Autodesk Inventor part; units mm, degrees
(part 6 of 16)
  spline S32 degree 3 poles (-26.5584, 48.5928) (-26.5078, 48.7178) (-26.4553, 48.842) (-26.4009, 48.9654) (-26.3715, 49.0321) (-26.3415, 49.0986) (-26.3109, 49.1648) (-26.2819, 49.2274) (-26.2524, 49.2898) (-26.2223, 49.3519) (-26.1939, 49.4105) (-26.165, 49.4689) (-26.1356, 49.527) (-26.1079, 49.5817) (-26.0798, 49.6361) (-26.0511, 49.6902) (-26.0243, 49.7409) (-25.997, 49.7914) (-25.9693, 49.8416) (-25.9435, 49.8884) (-25.9172, 49.935) (-25.8905, 49.9814) (-25.8658, 50.0244) (-25.8407, 50.0671) (-25.8152, 50.1097) (-25.7917, 50.1489) (-25.7679, 50.1879) (-25.7437, 50.2267) (-25.7216, 50.2622) (-25.6991, 50.2974) (-25.6764, 50.3325) (-25.6557, 50.3644) (-25.6348, 50.396) (-25.6136, 50.4275) (-25.5946, 50.4557) (-25.5753, 50.4838) (-25.5558, 50.5116) (-25.5299, 50.5485) (-25.5036, 50.5849) (-25.4769, 50.6212) (-25.4709, 50.6293) (-25.465, 50.6374) (-25.4591, 50.6456) (-25.4533, 50.6535) (-25.4476, 50.6616) (-25.442, 50.6697) (-25.4366, 50.6776) (-25.4311, 50.6855) (-25.4258, 50.6935) (-25.4205, 50.7014) (-25.4154, 50.7093) (-25.4103, 50.7172) (-25.4053, 50.725) (-25.4003, 50.7329) (-25.3955, 50.7408) (-25.3907, 50.7485) (-25.386, 50.7564) (-25.3815, 50.7642) (-25.3769, 50.772) (-25.3725, 50.7798) (-25.3681, 50.7877) (-25.3638, 50.7955) (-25.3596, 50.8034) (-25.3555, 50.8113) (-25.3514, 50.8192) (-25.3474, 50.8271) (-25.3435, 50.8351) (-25.3396, 50.8431) (-25.3358, 50.8512) (-25.3322, 50.8593) (-25.3285, 50.8675) (-25.3249, 50.8758) (-25.3215, 50.8841) (-25.3181, 50.8926) (-25.3148, 50.9011) (-25.3116, 50.9097) (-25.3084, 50.9185) (-25.3053, 50.9274) (-25.3024, 50.9364) (-25.2994, 50.9457) (-25.2967, 50.9551) (-25.2941, 50.9646) (-25.2914, 50.9746) (-25.289, 50.9846) (-25.2868, 50.9947) (-25.2845, 51.0055) (-25.2825, 51.0164) (-25.2808, 51.0274) (-25.279, 51.0393) (-25.2776, 51.0512) (-25.2767, 51.0632) (-25.2756, 51.0765) (-25.2751, 51.0897) (-25.2751, 51.103) (-25.2751, 51.1178) (-25.2759, 51.1326) (-25.2773, 51.1474) (-25.2789, 51.164) (-25.2815, 51.1804) (-25.2849, 51.1967) (-25.2888, 51.2151) (-25.2938, 51.2331) (-25.3, 51.2508) (-25.3069, 51.2704) (-25.3153, 51.2895) (-25.3249, 51.308) (-25.3354, 51.328) (-25.3475, 51.3472) (-25.3611, 51.3651) (-25.3742, 51.3822) (-25.3887, 51.3982) (-25.4035, 51.4138) (-25.4766, 51.4915) (-25.556, 51.5626) (-25.6317, 51.6374) (-25.7075, 51.7123) (-25.7795, 51.7908) (-25.858, 51.863) (-25.8739, 51.8776) (-25.89, 51.892) (-25.9072, 51.9048) (-25.9253, 51.9183) (-25.9447, 51.9301) (-25.9648, 51.9403) (-25.9833, 51.9498) (-26.0026, 51.9579) (-26.0223, 51.9646) (-26.04, 51.9706) (-26.0581, 51.9754) (-26.0765, 51.9791) (-26.0928, 51.9823) (-26.1093, 51.9847) (-26.1259, 51.9861) (-26.1407, 51.9874) (-26.1555, 51.9879) (-26.1703, 51.9878) (-26.1836, 51.9876) (-26.1969, 51.9869) (-26.2101, 51.9857) (-26.2221, 51.9846) (-26.234, 51.9831) (-26.2459, 51.9812) (-26.2568, 51.9794) (-26.2677, 51.9772) (-26.2785, 51.9748) (-26.2885, 51.9725) (-26.2986, 51.97) (-26.3085, 51.9672) (-26.318, 51.9645) (-26.3273, 51.9616) (-26.3366, 51.9585) (-26.3455, 51.9555) (-26.3544, 51.9524) (-26.3632, 51.949) (-26.3718, 51.9458) (-26.3802, 51.9423) (-26.3887, 51.9388) (-26.3969, 51.9353) (-26.4052, 51.9316) (-26.4133, 51.9279) (-26.4214, 51.9241) (-26.4294, 51.9202) (-26.4374, 51.9163) (-26.4453, 51.9123) (-26.4532, 51.9082) (-26.4611, 51.904) (-26.4689, 51.8998) (-26.4767, 51.8955) (-26.4845, 51.8911) (-26.4923, 51.8866) (-26.5001, 51.8821) (-26.5078, 51.8775) (-26.5156, 51.8728) (-26.5234, 51.868) (-26.5311, 51.8631) (-26.539, 51.8582) (-26.5468, 51.8532) (-26.5545, 51.8481) (-26.5624, 51.8429) (-26.5702, 51.8376) (-26.578, 51.8323) (-26.5859, 51.8269) (-26.5938, 51.8213) (-26.6017, 51.8158) (-26.6097, 51.8101) (-26.6177, 51.8043) (-26.6256, 51.7984) (-26.6337, 51.7925) (-26.6417, 51.7864) (-26.6497, 51.7803) (-26.6857, 51.7532) (-26.7218, 51.7265) (-26.7583, 51.7002) (-26.786, 51.6803) (-26.8138, 51.6607) (-26.8418, 51.6414) (-26.8731, 51.6198) (-26.9045, 51.5985) (-26.936, 51.5775) (-26.9708, 51.5543) (-27.0059, 51.5315) (-27.0411, 51.5089) (-27.0796, 51.4843) (-27.1183, 51.46) (-27.1572, 51.436) (-27.1995, 51.41) (-27.2419, 51.3844) (-27.2846, 51.3592) (-27.3307, 51.332) (-27.377, 51.3052) (-27.4235, 51.2788) (-27.4734, 51.2505) (-27.5235, 51.2227) (-27.5739, 51.1952) (-27.6277, 51.166) (-27.6818, 51.1372) (-27.7361, 51.1089) (-27.7938, 51.0788) (-27.8519, 51.0492) (-27.9102, 51.0201) (-27.9719, 50.9893) (-28.034, 50.959) (-28.0963, 50.9293) (-28.1621, 50.898) (-28.2282, 50.8672) (-28.2945, 50.837) (-28.4173, 50.7811) (-28.5409, 50.7272) (-28.6653, 50.6751) knots 0 0 0 0 0.057795 0.057795 0.057795 0.089038 0.089038 0.089038 0.118617 0.118617 0.118617 0.14653 0.14653 0.14653 0.172778 0.172778 0.172778 0.19736 0.19736 0.19736 0.220277 0.220277 0.220277 0.241529 0.241529 0.241529 0.261115 0.261115 0.261115 0.279036 0.279036 0.279036 0.295292 0.295292 0.295292 0.309882 0.309882 0.309882 0.329164 0.329164 0.329164 0.333477 0.333477 0.333477 0.337694 0.337694 0.337694 0.34182 0.34182 0.34182 0.345864 0.345864 0.345864 0.349834 0.349834 0.349834 0.353742 0.353742 0.353742 0.3576 0.3576 0.3576 0.361424 0.361424 0.361424 0.365232 0.365232 0.365232 0.369048 0.369048 0.369048 0.372899 0.372899 0.372899 0.376819 0.376819 0.376819 0.380853 0.380853 0.380853 0.385052 0.385052 0.385052 0.389482 0.389482 0.389482 0.394225 0.394225 0.394225 0.399381 0.399381 0.399381 0.405067 0.405067 0.405067 0.411413 0.411413 0.411413 0.418548 0.418548 0.418548 0.426565 0.426565 0.426565 0.435472 0.435472 0.435472 0.445133 0.445133 0.445133 0.45436 0.45436 0.45436 0.5 0.5 0.5 0.54564 0.54564 0.54564 0.554867 0.554867 0.554867 0.564528 0.564528 0.564528 0.573435 0.573435 0.573435 0.581452 0.581452 0.581452 0.588587 0.588587 0.588587 0.594933 0.594933 0.594933 0.600619 0.600619 0.600619 0.605775 0.605775 0.605775 0.610518 0.610518 0.610518 0.614948 0.614948 0.614948 0.619147 0.619147 0.619147 0.623181 0.623181 0.623181 0.627101 0.627101 0.627101 0.630952 0.630952 0.630952 0.634768 0.634768 0.634768 0.638576 0.638576 0.638576 0.6424 0.6424 0.6424 0.646258 0.646258 0.646258 0.650166 0.650166 0.650166 0.654136 0.654136 0.654136 0.65818 0.65818 0.65818 0.662306 0.662306 0.662306 0.666523 0.666523 0.666523 0.670836 0.670836 0.670836 0.690118 0.690118 0.690118 0.704708 0.704708 0.704708 0.720964 0.720964 0.720964 0.738885 0.738885 0.738885 0.758471 0.758471 0.758471 0.779723 0.779723 0.779723 0.80264 0.80264 0.80264 0.827222 0.827222 0.827222 0.85347 0.85347 0.85347 0.881383 0.881383 0.881383 0.910962 0.910962 0.910962 0.942205 0.942205 0.942205 1 1 1 1
  arc A234 (-26.5584, 48.5928) -> (-25.692, 47.8218) centre (0.0435, 77.6158) ccw
  spline S33 degree 3 poles (-23.379, 45.9711) (-23.3417, 46.1007) (-23.3025, 46.2298) (-23.2613, 46.3582) (-23.239, 46.4276) (-23.2161, 46.4968) (-23.1926, 46.5658) (-23.1703, 46.6312) (-23.1475, 46.6963) (-23.124, 46.7612) (-23.1019, 46.8225) (-23.0793, 46.8836) (-23.0561, 46.9444) (-23.0343, 47.0017) (-23.012, 47.0587) (-22.9891, 47.1156) (-22.9678, 47.1688) (-22.9459, 47.2218) (-22.9236, 47.2747) (-22.9028, 47.324) (-22.8816, 47.373) (-22.8599, 47.4219) (-22.8398, 47.4673) (-22.8193, 47.5124) (-22.7984, 47.5574) (-22.7791, 47.5988) (-22.7595, 47.6401) (-22.7395, 47.6812) (-22.7212, 47.7188) (-22.7026, 47.7563) (-22.6836, 47.7935) (-22.6664, 47.8273) (-22.6489, 47.861) (-22.6311, 47.8945) (-22.6151, 47.9246) (-22.5989, 47.9545) (-22.5824, 47.9843) (-22.5605, 48.0236) (-22.5381, 48.0626) (-22.5154, 48.1015) (-22.5103, 48.1101) (-22.5052, 48.1188) (-22.5002, 48.1276) (-22.4953, 48.1361) (-22.4905, 48.1447) (-22.4858, 48.1533) (-22.4812, 48.1617) (-22.4766, 48.1702) (-22.4721, 48.1787) (-22.4677, 48.1871) (-22.4634, 48.1955) (-22.4592, 48.2039) (-22.455, 48.2122) (-22.4509, 48.2205) (-22.4469, 48.2289) (-22.443, 48.2371) (-22.4392, 48.2454) (-22.4354, 48.2537) (-22.4317, 48.2619) (-22.4281, 48.2701) (-22.4246, 48.2784) (-22.4211, 48.2867) (-22.4178, 48.2949) (-22.4145, 48.3032) (-22.4112, 48.3115) (-22.4081, 48.3198) (-22.4051, 48.3282) (-22.402, 48.3365) (-22.3991, 48.345) (-22.3963, 48.3534) (-22.3935, 48.362) (-22.3909, 48.3705) (-22.3884, 48.3792) (-22.3858, 48.3879) (-22.3834, 48.3968) (-22.3812, 48.4056) (-22.3789, 48.4148) (-22.3767, 48.4239) (-22.3748, 48.4332) (-22.3728, 48.4428) (-22.371, 48.4524) (-22.3695, 48.4621) (-22.3679, 48.4723) (-22.3665, 48.4825) (-22.3654, 48.4928) (-22.3642, 48.5038) (-22.3634, 48.5149) (-22.3629, 48.5259) (-22.3623, 48.5379) (-22.3622, 48.55) (-22.3625, 48.562) (-22.3628, 48.5753) (-22.3637, 48.5885) (-22.3651, 48.6017) (-22.3667, 48.6165) (-22.3689, 48.6311) (-22.3719, 48.6456) (-22.3752, 48.6619) (-22.3795, 48.6781) (-22.3846, 48.6939) (-22.3904, 48.7117) (-22.3973, 48.7292) (-22.4053, 48.7461) (-22.4142, 48.7649) (-22.4245, 48.783) (-22.4361, 48.8003) (-22.4486, 48.8191) (-22.4626, 48.837) (-22.478, 48.8534) (-22.4928, 48.869) (-22.5089, 48.8834) (-22.5253, 48.8975) (-22.6061, 48.967) (-22.6925, 49.0295) (-22.7756, 49.096) (-22.8587, 49.1625) (-22.9386, 49.2331) (-23.0242, 49.2967) (-23.0415, 49.3095) (-23.059, 49.3221) (-23.0776, 49.3331) (-23.097, 49.3446) (-23.1174, 49.3543) (-23.1385, 49.3624) (-23.1579, 49.3698) (-23.1779, 49.3759) (-23.1982, 49.3805) (-23.2164, 49.3846) (-23.235, 49.3875) (-23.2536, 49.3892) (-23.2702, 49.3908) (-23.2869, 49.3914) (-23.3035, 49.391) (-23.3183, 49.3908) (-23.3331, 49.3898) (-23.3479, 49.3881) (-23.361, 49.3865) (-23.3742, 49.3845) (-23.3872, 49.3819) (-23.399, 49.3795) (-23.4107, 49.3768) (-23.4223, 49.3736) (-23.433, 49.3707) (-23.4436, 49.3674) (-23.4541, 49.3639) (-23.4639, 49.3606) (-23.4735, 49.357) (-23.4832, 49.3531) (-23.4923, 49.3495) (-23.5013, 49.3456) (-23.5102, 49.3416) (-23.5188, 49.3377) (-23.5272, 49.3336) (-23.5356, 49.3294) (-23.5438, 49.3252) (-23.5519, 49.3209) (-23.5599, 49.3165) (-23.5678, 49.3122) (-23.5756, 49.3077) (-23.5833, 49.3031) (-23.5909, 49.2985) (-23.5985, 49.2938) (-23.606, 49.289) (-23.6135, 49.2843) (-23.6209, 49.2794) (-23.6283, 49.2744) (-23.6356, 49.2694) (-23.643, 49.2643) (-23.6502, 49.2591) (-23.6575, 49.2538) (-23.6648, 49.2485) (-23.672, 49.2431) (-23.6793, 49.2376) (-23.6865, 49.232) (-23.6937, 49.2264) (-23.701, 49.2207) (-23.7082, 49.2149) (-23.7153, 49.209) (-23.7226, 49.203) (-23.7299, 49.197) (-23.7371, 49.1909) (-23.7444, 49.1846) (-23.7517, 49.1783) (-23.7589, 49.1719) (-23.7663, 49.1654) (-23.7736, 49.1588) (-23.7808, 49.1522) (-23.7883, 49.1454) (-23.7956, 49.1385) (-23.803, 49.1317) (-23.8359, 49.101) (-23.869, 49.0705) (-23.9026, 49.0406) (-23.928, 49.0179) (-23.9537, 48.9955) (-23.9795, 48.9734) (-24.0083, 48.9487) (-24.0373, 48.9242) (-24.0665, 48.9) (-24.0987, 48.8733) (-24.1311, 48.8469) (-24.1638, 48.8208) (-24.1995, 48.7923) (-24.2355, 48.7641) (-24.2717, 48.7362) (-24.311, 48.7059) (-24.3506, 48.676) (-24.3904, 48.6465) (-24.4333, 48.6146) (-24.4765, 48.5831) (-24.52, 48.552) (-24.5667, 48.5186) (-24.6137, 48.4857) (-24.6609, 48.4532) (-24.7114, 48.4184) (-24.7621, 48.3842) (-24.8132, 48.3503) (-24.8675, 48.3143) (-24.9221, 48.2789) (-24.977, 48.2438) (-25.0352, 48.2067) (-25.0938, 48.1702) (-25.1526, 48.1341) (-25.2148, 48.096) (-25.2773, 48.0585) (-25.3402, 48.0215) (-25.4564, 47.9531) (-25.5737, 47.8866) (-25.692, 47.8218) knots 0 0 0 0 0.057795 0.057795 0.057795 0.089038 0.089038 0.089038 0.118617 0.118617 0.118617 0.14653 0.14653 0.14653 0.172778 0.172778 0.172778 0.19736 0.19736 0.19736 0.220277 0.220277 0.220277 0.241529 0.241529 0.241529 0.261115 0.261115 0.261115 0.279036 0.279036 0.279036 0.295292 0.295292 0.295292 0.309882 0.309882 0.309882 0.329164 0.329164 0.329164 0.333477 0.333477 0.333477 0.337694 0.337694 0.337694 0.34182 0.34182 0.34182 0.345864 0.345864 0.345864 0.349834 0.349834 0.349834 0.353742 0.353742 0.353742 0.3576 0.3576 0.3576 0.361424 0.361424 0.361424 0.365232 0.365232 0.365232 0.369048 0.369048 0.369048 0.372899 0.372899 0.372899 0.376819 0.376819 0.376819 0.380853 0.380853 0.380853 0.385052 0.385052 0.385052 0.389482 0.389482 0.389482 0.394225 0.394225 0.394225 0.399381 0.399381 0.399381 0.405067 0.405067 0.405067 0.411413 0.411413 0.411413 0.418548 0.418548 0.418548 0.426565 0.426565 0.426565 0.435472 0.435472 0.435472 0.445133 0.445133 0.445133 0.45436 0.45436 0.45436 0.5 0.5 0.5 0.54564 0.54564 0.54564 0.554867 0.554867 0.554867 0.564528 0.564528 0.564528 0.573435 0.573435 0.573435 0.581452 0.581452 0.581452 0.588587 0.588587 0.588587 0.594933 0.594933 0.594933 0.600619 0.600619 0.600619 0.605775 0.605775 0.605775 0.610518 0.610518 0.610518 0.614948 0.614948 0.614948 0.619147 0.619147 0.619147 0.623181 0.623181 0.623181 0.627101 0.627101 0.627101 0.630952 0.630952 0.630952 0.634768 0.634768 0.634768 0.638576 0.638576 0.638576 0.6424 0.6424 0.6424 0.646258 0.646258 0.646258 0.650166 0.650166 0.650166 0.654136 0.654136 0.654136 0.65818 0.65818 0.65818 0.662306 0.662306 0.662306 0.666523 0.666523 0.666523 0.670836 0.670836 0.670836 0.690118 0.690118 0.690118 0.704708 0.704708 0.704708 0.720964 0.720964 0.720964 0.738885 0.738885 0.738885 0.758471 0.758471 0.758471 0.779723 0.779723 0.779723 0.80264 0.80264 0.80264 0.827222 0.827222 0.827222 0.85347 0.85347 0.85347 0.881383 0.881383 0.881383 0.910962 0.910962 0.910962 0.942205 0.942205 0.942205 1 1 1 1
  arc A235 (-23.379, 45.9711) -> (-22.4367, 45.2949) centre (0.0435, 77.6158) ccw
  spline S34 degree 3 poles (-19.9429, 43.6961) (-19.9194, 43.8289) (-19.8939, 43.9614) (-19.8663, 44.0934) (-19.8514, 44.1648) (-19.8358, 44.236) (-19.8197, 44.3071) (-19.8043, 44.3744) (-19.7884, 44.4416) (-19.7719, 44.5086) (-19.7563, 44.5718) (-19.7402, 44.6349) (-19.7235, 44.6979) (-19.7078, 44.7571) (-19.6916, 44.8162) (-19.6748, 44.8751) (-19.6591, 44.9303) (-19.643, 44.9853) (-19.6263, 45.0402) (-19.6107, 45.0914) (-19.5948, 45.1424) (-19.5783, 45.1933) (-19.5631, 45.2405) (-19.5474, 45.2875) (-19.5313, 45.3344) (-19.5165, 45.3777) (-19.5013, 45.4208) (-19.4857, 45.4637) (-19.4714, 45.503) (-19.4568, 45.5422) (-19.4418, 45.5813) (-19.4283, 45.6167) (-19.4144, 45.652) (-19.4002, 45.6872) (-19.3874, 45.7187) (-19.3744, 45.7502) (-19.3611, 45.7815) (-19.3435, 45.8229) (-19.3253, 45.8641) (-19.3067, 45.9051) (-19.3026, 45.9143) (-19.2984, 45.9234) (-19.2944, 45.9326) (-19.2904, 45.9416) (-19.2865, 45.9507) (-19.2827, 45.9598) (-19.279, 45.9686) (-19.2753, 45.9775) (-19.2718, 45.9865) (-19.2683, 45.9952) (-19.2648, 46.004) (-19.2615, 46.0129) (-19.2582, 46.0215) (-19.2551, 46.0302) (-19.252, 46.039) (-19.2489, 46.0476) (-19.246, 46.0562) (-19.2431, 46.0649) (-19.2403, 46.0734) (-19.2376, 46.082) (-19.2349, 46.0906) (-19.2323, 46.0991) (-19.2298, 46.1077) (-19.2275, 46.1163) (-19.2251, 46.1249) (-19.2228, 46.1335) (-19.2207, 46.1421) (-19.2186, 46.1507) (-19.2165, 46.1594) (-19.2147, 46.1681) (-19.2128, 46.1769) (-19.211, 46.1857) (-19.2094, 46.1946) (-19.2078, 46.2036) (-19.2063, 46.2126) (-19.205, 46.2217) (-19.2037, 46.231) (-19.2025, 46.2403) (-19.2016, 46.2497) (-19.2006, 46.2594) (-19.1998, 46.2692) (-19.1993, 46.279) (-19.1988, 46.2893) (-19.1985, 46.2996) (-19.1984, 46.31) (-19.1984, 46.3211) (-19.1987, 46.3321) (-19.1994, 46.3432) (-19.2001, 46.3552) (-19.2012, 46.3672) (-19.2028, 46.3791) (-19.2045, 46.3923) (-19.2067, 46.4054) (-19.2095, 46.4183) (-19.2126, 46.4328) (-19.2164, 46.4472) (-19.2209, 46.4613) (-19.2259, 46.4772) (-19.2318, 46.4928) (-19.2386, 46.508) (-19.2462, 46.5251) (-19.2549, 46.5417) (-19.2646, 46.5577) (-19.2755, 46.5755) (-19.2876, 46.5924) (-19.3009, 46.6084) (-19.3153, 46.6258) (-19.3311, 46.6421) (-19.3482, 46.6568) (-19.3645, 46.6708) (-19.382, 46.6834) (-19.3997, 46.6957) (-19.4874, 46.7564) (-19.5798, 46.8095) (-19.6695, 46.867) (-19.7591, 46.9244) (-19.8459, 46.9863) (-19.9377, 47.0406) (-19.9562, 47.0516) (-19.975, 47.0622) (-19.9946, 47.0712) (-20.015, 47.0806) (-20.0364, 47.0881) (-20.0582, 47.094) (-20.0783, 47.0994) (-20.0988, 47.1033) (-20.1195, 47.1057) (-20.1381, 47.1079) (-20.1568, 47.1089) (-20.1755, 47.1087) (-20.1922, 47.1084) (-20.2088, 47.1073) (-20.2253, 47.1052) (-20.24, 47.1034) (-20.2547, 47.1009) (-20.2691, 47.0976) (-20.2821, 47.0947) (-20.2949, 47.0913) (-20.3076, 47.0874) (-20.3191, 47.0838) (-20.3304, 47.0798) (-20.3416, 47.0755) (-20.352, 47.0715) (-20.3622, 47.0671) (-20.3722, 47.0625) (-20.3816, 47.0582) (-20.3909, 47.0536) (-20.4, 47.0487) (-20.4087, 47.0442) (-20.4172, 47.0394) (-20.4257, 47.0344) (-20.4338, 47.0297) (-20.4418, 47.0247) (-20.4497, 47.0196) (-20.4574, 47.0147) (-20.465, 47.0096) (-20.4725, 47.0043) (-20.4799, 46.9992) (-20.4872, 46.9939) (-20.4944, 46.9885) (-20.5015, 46.9832) (-20.5085, 46.9777) (-20.5155, 46.9722) (-20.5224, 46.9666) (-20.5293, 46.961) (-20.5361, 46.9553) (-20.5429, 46.9495) (-20.5497, 46.9437) (-20.5563, 46.9377) (-20.5631, 46.9318) (-20.5697, 46.9257) (-20.5763, 46.9196) (-20.583, 46.9134) (-20.5896, 46.9071) (-20.5961, 46.9007) (-20.6028, 46.8943) (-20.6094, 46.8877) (-20.6159, 46.8811) (-20.6225, 46.8744) (-20.6291, 46.8677) (-20.6356, 46.8608) (-20.6422, 46.8538) (-20.6488, 46.8468) (-20.6553, 46.8397) (-20.662, 46.8325) (-20.6686, 46.8252) (-20.6751, 46.8178) (-20.6817, 46.8103) (-20.6883, 46.8027) (-20.6949, 46.7951) (-20.7245, 46.7611) (-20.7542, 46.7274) (-20.7845, 46.6941) (-20.8074, 46.6689) (-20.8306, 46.6439) (-20.854, 46.6192) (-20.88, 46.5916) (-20.9063, 46.5642) (-20.9328, 46.5371) (-20.962, 46.5072) (-20.9915, 46.4776) (-21.0213, 46.4482) (-21.0538, 46.4161) (-21.0867, 46.3843) (-21.1198, 46.3528) (-21.1557, 46.3186) (-21.1919, 46.2847) (-21.2284, 46.2511) (-21.2678, 46.215) (-21.3075, 46.1791) (-21.3475, 46.1436) (-21.3904, 46.1056) (-21.4337, 46.0679) (-21.4773, 46.0306) (-21.5238, 45.9908) (-21.5707, 45.9514) (-21.6179, 45.9124) (-21.6682, 45.871) (-21.7188, 45.83) (-21.7698, 45.7894) (-21.8238, 45.7464) (-21.8782, 45.7039) (-21.9329, 45.6619) (-21.9908, 45.6175) (-22.049, 45.5737) (-22.1077, 45.5303) (-22.2161, 45.4502) (-22.3258, 45.3717) (-22.4367, 45.2949) knots 0 0 0 0 0.057795 0.057795 0.057795 0.089038 0.089038 0.089038 0.118617 0.118617 0.118617 0.14653 0.14653 0.14653 0.172778 0.172778 0.172778 0.19736 0.19736 0.19736 0.220277 0.220277 0.220277 0.241529 0.241529 0.241529 0.261115 0.261115 0.261115 0.279036 0.279036 0.279036 0.295292 0.295292 0.295292 0.309882 0.309882 0.309882 0.329164 0.329164 0.329164 0.333477 0.333477 0.333477 0.337694 0.337694 0.337694 0.34182 0.34182 0.34182 0.345864 0.345864 0.345864 0.349834 0.349834 0.349834 0.353742 0.353742 0.353742 0.3576 0.3576 0.3576 0.361424 0.361424 0.361424 0.365232 0.365232 0.365232 0.369048 0.369048 0.369048 0.372899 0.372899 0.372899 0.376819 0.376819 0.376819 0.380853 0.380853 0.380853 0.385052 0.385052 0.385052 0.389482 0.389482 0.389482 0.394225 0.394225 0.394225 0.399381 0.399381 0.399381 0.405067 0.405067 0.405067 0.411413 0.411413 0.411413 0.418548 0.418548 0.418548 0.426565 0.426565 0.426565 0.435472 0.435472 0.435472 0.445133 0.445133 0.445133 0.45436 0.45436 0.45436 0.5 0.5 0.5 0.54564 0.54564 0.54564 0.554867 0.554867 0.554867 0.564528 0.564528 0.564528 0.573435 0.573435 0.573435 0.581452 0.581452 0.581452 0.588587 0.588587 0.588587 0.594933 0.594933 0.594933 0.600619 0.600619 0.600619 0.605775 0.605775 0.605775 0.610518 0.610518 0.610518 0.614948 0.614948 0.614948 0.619147 0.619147 0.619147 0.623181 0.623181 0.623181 0.627101 0.627101 0.627101 0.630952 0.630952 0.630952 0.634768 0.634768 0.634768 0.638576 0.638576 0.638576 0.6424 0.6424 0.6424 0.646258 0.646258 0.646258 0.650166 0.650166 0.650166 0.654136 0.654136 0.654136 0.65818 0.65818 0.65818 0.662306 0.662306 0.662306 0.666523 0.666523 0.666523 0.670836 0.670836 0.670836 0.690118 0.690118 0.690118 0.704708 0.704708 0.704708 0.720964 0.720964 0.720964 0.738885 0.738885 0.738885 0.758471 0.758471 0.758471 0.779723 0.779723 0.779723 0.80264 0.80264 0.80264 0.827222 0.827222 0.827222 0.85347 0.85347 0.85347 0.881383 0.881383 0.881383 0.910962 0.910962 0.910962 0.942205 0.942205 0.942205 1 1 1 1
  arc A236 (-19.9429, 43.6961) -> (-18.9351, 43.1221) centre (0.0435, 77.6158) ccw
  spline S35 degree 3 poles (-16.2878, 41.7928) (-16.2783, 41.9273) (-16.2668, 42.0617) (-16.2532, 42.1959) (-16.2458, 42.2684) (-16.2378, 42.3409) (-16.2291, 42.4133) (-16.2209, 42.4818) (-16.2122, 42.5503) (-16.2027, 42.6187) (-16.1939, 42.6832) (-16.1844, 42.7477) (-16.1744, 42.812) (-16.1649, 42.8725) (-16.155, 42.933) (-16.1445, 42.9933) (-16.1346, 43.0498) (-16.1243, 43.1063) (-16.1135, 43.1626) (-16.1034, 43.2151) (-16.0928, 43.2675) (-16.0818, 43.3199) (-16.0715, 43.3684) (-16.0609, 43.4168) (-16.0498, 43.4651) (-16.0395, 43.5097) (-16.0289, 43.5541) (-16.0179, 43.5985) (-16.0078, 43.6391) (-15.9974, 43.6796) (-15.9866, 43.72) (-15.9768, 43.7566) (-15.9667, 43.7932) (-15.9562, 43.8297) (-15.9468, 43.8624) (-15.9372, 43.8951) (-15.9272, 43.9276) (-15.914, 43.9706) (-15.9002, 44.0134) (-15.8861, 44.0562) (-15.8829, 44.0657) (-15.8797, 44.0753) (-15.8766, 44.0848) (-15.8736, 44.0942) (-15.8707, 44.1036) (-15.8679, 44.113) (-15.8651, 44.1222) (-15.8624, 44.1315) (-15.8598, 44.1408) (-15.8572, 44.1498) (-15.8547, 44.1589) (-15.8524, 44.1681) (-15.85, 44.177) (-15.8478, 44.186) (-15.8456, 44.195) (-15.8435, 44.2039) (-15.8414, 44.2128) (-15.8395, 44.2217) (-15.8376, 44.2305) (-15.8358, 44.2393) (-15.834, 44.2482) (-15.8324, 44.2569) (-15.8308, 44.2657) (-15.8293, 44.2745) (-15.8278, 44.2833) (-15.8265, 44.292) (-15.8253, 44.3009) (-15.824, 44.3097) (-15.823, 44.3185) (-15.822, 44.3274) (-15.821, 44.3363) (-15.8202, 44.3452) (-15.8195, 44.3542) (-15.8189, 44.3633) (-15.8183, 44.3725) (-15.818, 44.3816) (-15.8177, 44.391) (-15.8175, 44.4004) (-15.8175, 44.4098) (-15.8176, 44.4196) (-15.8178, 44.4294) (-15.8183, 44.4392) (-15.8188, 44.4496) (-15.8196, 44.4599) (-15.8207, 44.4702) (-15.8218, 44.4812) (-15.8233, 44.4921) (-15.8251, 44.5031) (-15.8271, 44.5149) (-15.8294, 44.5267) (-15.8322, 44.5384) (-15.8353, 44.5514) (-15.8389, 44.5641) (-15.843, 44.5768) (-15.8476, 44.5908) (-15.8529, 44.6047) (-15.8588, 44.6183) (-15.8655, 44.6335) (-15.873, 44.6484) (-15.8813, 44.6629) (-15.8907, 44.6791) (-15.9011, 44.6947) (-15.9124, 44.7096) (-15.925, 44.7261) (-15.9389, 44.7417) (-15.9538, 44.7563) (-15.9699, 44.772) (-15.9873, 44.7866) (-16.0058, 44.7994) (-16.0235, 44.8117) (-16.0423, 44.8224) (-16.0612, 44.8327) (-16.1547, 44.8839) (-16.2522, 44.9271) (-16.3473, 44.9748) (-16.4425, 45.0226) (-16.5353, 45.0751) (-16.6322, 45.1195) (-16.6518, 45.1284) (-16.6716, 45.1371) (-16.692, 45.144) (-16.7134, 45.1512) (-16.7354, 45.1564) (-16.7577, 45.16) (-16.7783, 45.1632) (-16.7991, 45.165) (-16.8198, 45.1653) (-16.8386, 45.1655) (-16.8573, 45.1645) (-16.8759, 45.1623) (-16.8924, 45.1604) (-16.9089, 45.1575) (-16.9251, 45.1537) (-16.9395, 45.1503) (-16.9538, 45.1463) (-16.9678, 45.1416) (-16.9804, 45.1373) (-16.9928, 45.1326) (-17.005, 45.1274) (-17.0161, 45.1226) (-17.0269, 45.1175) (-17.0376, 45.1119) (-17.0475, 45.1069) (-17.0572, 45.1015) (-17.0667, 45.0958) (-17.0756, 45.0905) (-17.0843, 45.085) (-17.0929, 45.0793) (-17.101, 45.0738) (-17.1091, 45.0682) (-17.1169, 45.0624) (-17.1245, 45.0568) (-17.132, 45.051) (-17.1393, 45.0451) (-17.1464, 45.0394) (-17.1534, 45.0335) (-17.1604, 45.0275) (-17.1672, 45.0216) (-17.1738, 45.0156) (-17.1804, 45.0095) (-17.187, 45.0035) (-17.1934, 44.9973) (-17.1997, 44.991) (-17.2061, 44.9848) (-17.2123, 44.9785) (-17.2185, 44.9721) (-17.2246, 44.9656) (-17.2307, 44.9591) (-17.2368, 44.9525) (-17.2428, 44.9459) (-17.2488, 44.9392) (-17.2547, 44.9324) (-17.2607, 44.9255) (-17.2666, 44.9186) (-17.2725, 44.9116) (-17.2784, 44.9044) (-17.2843, 44.8973) (-17.2901, 44.89) (-17.2959, 44.8827) (-17.3018, 44.8752) (-17.3075, 44.8677) (-17.3134, 44.8601) (-17.3192, 44.8524) (-17.3249, 44.8447) (-17.3308, 44.8368) (-17.3366, 44.8288) (-17.3423, 44.8208) (-17.3482, 44.8126) (-17.3539, 44.8044) (-17.3597, 44.7961) (-17.3855, 44.7593) (-17.4116, 44.7226) (-17.4382, 44.6864) (-17.4584, 44.6589) (-17.4788, 44.6317) (-17.4995, 44.6046) (-17.5225, 44.5745) (-17.5457, 44.5445) (-17.5693, 44.5148) (-17.5952, 44.482) (-17.6215, 44.4494) (-17.648, 44.4171) (-17.677, 44.3818) (-17.7063, 44.3467) (-17.736, 44.3119) (-17.7681, 44.2741) (-17.8006, 44.2366) (-17.8334, 44.1994) (-17.8688, 44.1593) (-17.9045, 44.1196) (-17.9406, 44.0801) (-17.9793, 44.0377) (-18.0184, 43.9958) (-18.0578, 43.9541) (-18.0999, 43.9096) (-18.1425, 43.8656) (-18.1854, 43.8219) (-18.231, 43.7754) (-18.2771, 43.7293) (-18.3235, 43.6836) (-18.3727, 43.6352) (-18.4224, 43.5873) (-18.4725, 43.5398) (-18.5253, 43.4896) (-18.5787, 43.4399) (-18.6325, 43.3907) (-18.7319, 43.2996) (-18.8329, 43.2101) (-18.9351, 43.1221) knots 0 0 0 0 0.057795 0.057795 0.057795 0.089038 0.089038 0.089038 0.118617 0.118617 0.118617 0.14653 0.14653 0.14653 0.172778 0.172778 0.172778 0.19736 0.19736 0.19736 0.220277 0.220277 0.220277 0.241529 0.241529 0.241529 0.261115 0.261115 0.261115 0.279036 0.279036 0.279036 0.295292 0.295292 0.295292 0.309882 0.309882 0.309882 0.329164 0.329164 0.329164 0.333477 0.333477 0.333477 0.337694 0.337694 0.337694 0.34182 0.34182 0.34182 0.345864 0.345864 0.345864 0.349834 0.349834 0.349834 0.353742 0.353742 0.353742 0.3576 0.3576 0.3576 0.361424 0.361424 0.361424 0.365232 0.365232 0.365232 0.369048 0.369048 0.369048 0.372899 0.372899 0.372899 0.376819 0.376819 0.376819 0.380853 0.380853 0.380853 0.385052 0.385052 0.385052 0.389482 0.389482 0.389482 0.394225 0.394225 0.394225 0.399381 0.399381 0.399381 0.405067 0.405067 0.405067 0.411413 0.411413 0.411413 0.418548 0.418548 0.418548 0.426565 0.426565 0.426565 0.435472 0.435472 0.435472 0.445133 0.445133 0.445133 0.45436 0.45436 0.45436 0.5 0.5 0.5 0.54564 0.54564 0.54564 0.554867 0.554867 0.554867 0.564528 0.564528 0.564528 0.573435 0.573435 0.573435 0.581452 0.581452 0.581452 0.588587 0.588587 0.588587 0.594933 0.594933 0.594933 0.600619 0.600619 0.600619 0.605775 0.605775 0.605775 0.610518 0.610518 0.610518 0.614948 0.614948 0.614948 0.619147 0.619147 0.619147 0.623181 0.623181 0.623181 0.627101 0.627101 0.627101 0.630952 0.630952 0.630952 0.634768 0.634768 0.634768 0.638576 0.638576 0.638576 0.6424 0.6424 0.6424 0.646258 0.646258 0.646258 0.650166 0.650166 0.650166 0.654136 0.654136 0.654136 0.65818 0.65818 0.65818 0.662306 0.662306 0.662306 0.666523 0.666523 0.666523 0.670836 0.670836 0.670836 0.690118 0.690118 0.690118 0.704708 0.704708 0.704708 0.720964 0.720964 0.720964 0.738885 0.738885 0.738885 0.758471 0.758471 0.758471 0.779723 0.779723 0.779723 0.80264 0.80264 0.80264 0.827222 0.827222 0.827222 0.85347 0.85347 0.85347 0.881383 0.881383 0.881383 0.910962 0.910962 0.910962 0.942205 0.942205 0.942205 1 1 1 1
  arc A237 (-16.2878, 41.7928) -> (-15.2255, 41.3273) centre (0.0435, 77.6158) ccw
  spline S36 degree 3 poles (-12.4539, 40.282) (-12.4584, 40.4168) (-12.4611, 40.5516) (-12.4615, 40.6865) (-12.4618, 40.7594) (-12.4614, 40.8323) (-12.4603, 40.9052) (-12.4594, 40.9742) (-12.4578, 41.0432) (-12.4555, 41.1122) (-12.4535, 41.1773) (-12.4508, 41.2424) (-12.4475, 41.3074) (-12.4445, 41.3686) (-12.4409, 41.4298) (-12.4368, 41.4909) (-12.4329, 41.5481) (-12.4285, 41.6053) (-12.4236, 41.6625) (-12.419, 41.7157) (-12.414, 41.769) (-12.4085, 41.8222) (-12.4034, 41.8715) (-12.3979, 41.9208) (-12.3919, 41.97) (-12.3864, 42.0154) (-12.3805, 42.0607) (-12.3741, 42.106) (-12.3683, 42.1474) (-12.3622, 42.1888) (-12.3557, 42.2301) (-12.3498, 42.2675) (-12.3435, 42.305) (-12.337, 42.3423) (-12.3311, 42.3759) (-12.3249, 42.4093) (-12.3184, 42.4428) (-12.3097, 42.4869) (-12.3005, 42.5309) (-12.2909, 42.5749) (-12.2887, 42.5847) (-12.2866, 42.5946) (-12.2845, 42.6044) (-12.2825, 42.614) (-12.2806, 42.6237) (-12.2787, 42.6334) (-12.2769, 42.6428) (-12.2752, 42.6523) (-12.2736, 42.6618) (-12.272, 42.6711) (-12.2705, 42.6804) (-12.269, 42.6897) (-12.2676, 42.6989) (-12.2663, 42.7081) (-12.2651, 42.7173) (-12.2639, 42.7263) (-12.2628, 42.7353) (-12.2618, 42.7444) (-12.2609, 42.7534) (-12.26, 42.7623) (-12.2592, 42.7713) (-12.2584, 42.7802) (-12.2578, 42.7891) (-12.2572, 42.798) (-12.2567, 42.8069) (-12.2563, 42.8157) (-12.256, 42.8246) (-12.2557, 42.8335) (-12.2555, 42.8424) (-12.2555, 42.8513) (-12.2555, 42.8603) (-12.2556, 42.8693) (-12.2559, 42.8783) (-12.2561, 42.8874) (-12.2566, 42.8966) (-12.2572, 42.9057) (-12.2578, 42.9151) (-12.2586, 42.9245) (-12.2597, 42.9338) (-12.2607, 42.9436) (-12.262, 42.9533) (-12.2635, 42.963) (-12.2651, 42.9732) (-12.267, 42.9834) (-12.2691, 42.9935) (-12.2714, 43.0043) (-12.274, 43.0151) (-12.277, 43.0257) (-12.2802, 43.0373) (-12.2837, 43.0488) (-12.2878, 43.0602) (-12.2922, 43.0727) (-12.2971, 43.085) (-12.3025, 43.0972) (-12.3085, 43.1107) (-12.3152, 43.1239) (-12.3225, 43.1368) (-12.3308, 43.1513) (-12.3398, 43.1653) (-12.3496, 43.1788) (-12.3606, 43.194) (-12.3725, 43.2084) (-12.3854, 43.222) (-12.3997, 43.2371) (-12.415, 43.2512) (-12.4314, 43.2641) (-12.4491, 43.2781) (-12.4679, 43.2908) (-12.4877, 43.3016) (-12.5066, 43.3119) (-12.5263, 43.3206) (-12.5462, 43.3289) (-12.6446, 43.3701) (-12.746, 43.4028) (-12.8457, 43.4403) (-12.9453, 43.4779) (-13.0431, 43.5204) (-13.1441, 43.5544) (-13.1645, 43.5613) (-13.1851, 43.5678) (-13.2061, 43.5725) (-13.2281, 43.5775) (-13.2506, 43.5804) (-13.2731, 43.5816) (-13.2939, 43.5827) (-13.3148, 43.5823) (-13.3355, 43.5803) (-13.3541, 43.5786) (-13.3726, 43.5757) (-13.3909, 43.5715) (-13.4071, 43.5679) (-13.4232, 43.5633) (-13.4389, 43.5578) (-13.4529, 43.553) (-13.4667, 43.5475) (-13.4802, 43.5413) (-13.4922, 43.5358) (-13.5041, 43.5298) (-13.5156, 43.5233) (-13.5261, 43.5174) (-13.5364, 43.5111) (-13.5465, 43.5045) (-13.5558, 43.4985) (-13.5648, 43.4921) (-13.5737, 43.4855) (-13.582, 43.4793) (-13.5901, 43.4729) (-13.598, 43.4663) (-13.6056, 43.46) (-13.6129, 43.4535) (-13.6202, 43.4469) (-13.6271, 43.4406) (-13.6339, 43.4341) (-13.6406, 43.4274) (-13.6471, 43.421) (-13.6535, 43.4144) (-13.6597, 43.4077) (-13.6659, 43.4012) (-13.6719, 43.3945) (-13.6778, 43.3877) (-13.6837, 43.381) (-13.6894, 43.3742) (-13.6951, 43.3674) (-13.7007, 43.3605) (-13.7063, 43.3536) (-13.7117, 43.3465) (-13.7172, 43.3395) (-13.7226, 43.3324) (-13.7279, 43.3252) (-13.7332, 43.3179) (-13.7385, 43.3106) (-13.7436, 43.3033) (-13.7489, 43.2958) (-13.754, 43.2883) (-13.7591, 43.2807) (-13.7643, 43.273) (-13.7693, 43.2652) (-13.7743, 43.2574) (-13.7794, 43.2495) (-13.7844, 43.2415) (-13.7894, 43.2335) (-13.7944, 43.2253) (-13.7994, 43.217) (-13.8043, 43.2087) (-13.8093, 43.2003) (-13.8142, 43.1917) (-13.8191, 43.1832) (-13.824, 43.1744) (-13.8289, 43.1656) (-13.8338, 43.1568) (-13.8556, 43.1174) (-13.8777, 43.0783) (-13.9004, 43.0394) (-13.9175, 43.01) (-13.935, 42.9808) (-13.9527, 42.9517) (-13.9725, 42.9193) (-13.9925, 42.8871) (-14.0128, 42.855) (-14.0352, 42.8197) (-14.0579, 42.7846) (-14.0809, 42.7497) (-14.106, 42.7115) (-14.1315, 42.6736) (-14.1574, 42.6359) (-14.1854, 42.5949) (-14.2138, 42.5543) (-14.2425, 42.5139) (-14.2735, 42.4703) (-14.3049, 42.427) (-14.3366, 42.3839) (-14.3707, 42.3378) (-14.4052, 42.292) (-14.4401, 42.2464) (-14.4773, 42.1978) (-14.515, 42.1495) (-14.5531, 42.1015) (-14.5936, 42.0505) (-14.6346, 41.9999) (-14.676, 41.9496) (-14.7199, 41.8964) (-14.7643, 41.8435) (-14.8091, 41.791) (-14.8565, 41.7356) (-14.9043, 41.6806) (-14.9527, 41.626) (-15.0421, 41.525) (-15.1331, 41.4255) (-15.2255, 41.3273) knots 0 0 0 0 0.057795 0.057795 0.057795 0.089038 0.089038 0.089038 0.118617 0.118617 0.118617 0.14653 0.14653 0.14653 0.172778 0.172778 0.172778 0.19736 0.19736 0.19736 0.220277 0.220277 0.220277 0.241529 0.241529 0.241529 0.261115 0.261115 0.261115 0.279036 0.279036 0.279036 0.295292 0.295292 0.295292 0.309882 0.309882 0.309882 0.329164 0.329164 0.329164 0.333477 0.333477 0.333477 0.337694 0.337694 0.337694 0.34182 0.34182 0.34182 0.345864 0.345864 0.345864 0.349834 0.349834 0.349834 0.353742 0.353742 0.353742 0.3576 0.3576 0.3576 0.361424 0.361424 0.361424 0.365232 0.365232 0.365232 0.369048 0.369048 0.369048 0.372899 0.372899 0.372899 0.376819 0.376819 0.376819 0.380853 0.380853 0.380853 0.385052 0.385052 0.385052 0.389482 0.389482 0.389482 0.394225 0.394225 0.394225 0.399381 0.399381 0.399381 0.405067 0.405067 0.405067 0.411413 0.411413 0.411413 0.418548 0.418548 0.418548 0.426565 0.426565 0.426565 0.435472 0.435472 0.435472 0.445133 0.445133 0.445133 0.45436 0.45436 0.45436 0.5 0.5 0.5 0.54564 0.54564 0.54564 0.554867 0.554867 0.554867 0.564528 0.564528 0.564528 0.573435 0.573435 0.573435 0.581452 0.581452 0.581452 0.588587 0.588587 0.588587 0.594933 0.594933 0.594933 0.600619 0.600619 0.600619 0.605775 0.605775 0.605775 0.610518 0.610518 0.610518 0.614948 0.614948 0.614948 0.619147 0.619147 0.619147 0.623181 0.623181 0.623181 0.627101 0.627101 0.627101 0.630952 0.630952 0.630952 0.634768 0.634768 0.634768 0.638576 0.638576 0.638576 0.6424 0.6424 0.6424 0.646258 0.646258 0.646258 0.650166 0.650166 0.650166 0.654136 0.654136 0.654136 0.65818 0.65818 0.65818 0.662306 0.662306 0.662306 0.666523 0.666523 0.666523 0.670836 0.670836 0.670836 0.690118 0.690118 0.690118 0.704708 0.704708 0.704708 0.720964 0.720964 0.720964 0.738885 0.738885 0.738885 0.758471 0.758471 0.758471 0.779723 0.779723 0.779723 0.80264 0.80264 0.80264 0.827222 0.827222 0.827222 0.85347 0.85347 0.85347 0.881383 0.881383 0.881383 0.910962 0.910962 0.910962 0.942205 0.942205 0.942205 1 1 1 1
  arc A238 (-12.4539, 40.282) -> (-11.3487, 39.93) centre (0.0435, 77.6158) ccw
  spline S37 degree 3 poles (-8.4829, 39.1802) (-8.5016, 39.3137) (-8.5183, 39.4476) (-8.5329, 39.5816) (-8.5407, 39.6541) (-8.548, 39.7267) (-8.5545, 39.7993) (-8.5608, 39.868) (-8.5664, 39.9368) (-8.5714, 40.0057) (-8.5761, 40.0706) (-8.5803, 40.1356) (-8.5839, 40.2007) (-8.5872, 40.2618) (-8.5901, 40.323) (-8.5923, 40.3842) (-8.5944, 40.4416) (-8.5961, 40.4989) (-8.5972, 40.5563) (-8.5982, 40.6097) (-8.5988, 40.6632) (-8.5989, 40.7167) (-8.5989, 40.7663) (-8.5986, 40.8159) (-8.5978, 40.8654) (-8.597, 40.9111) (-8.5959, 40.9568) (-8.5943, 41.0025) (-8.5929, 41.0443) (-8.5911, 41.0861) (-8.589, 41.1279) (-8.587, 41.1657) (-8.5847, 41.2036) (-8.5821, 41.2414) (-8.5797, 41.2754) (-8.5771, 41.3094) (-8.5741, 41.3433) (-8.5701, 41.3881) (-8.5655, 41.4328) (-8.5605, 41.4776) (-8.5594, 41.4876) (-8.5583, 41.4976) (-8.5573, 41.5076) (-8.5563, 41.5174) (-8.5554, 41.5272) (-8.5546, 41.537) (-8.5538, 41.5466) (-8.553, 41.5562) (-8.5524, 41.5658) (-8.5518, 41.5752) (-8.5513, 41.5846) (-8.5508, 41.5941) (-8.5504, 41.6033) (-8.5501, 41.6126) (-8.5498, 41.6218) (-8.5496, 41.6309) (-8.5494, 41.6401) (-8.5494, 41.6492) (-8.5493, 41.6582) (-8.5494, 41.6672) (-8.5496, 41.6762) (-8.5497, 41.6851) (-8.55, 41.694) (-8.5504, 41.7029) (-8.5508, 41.7118) (-8.5513, 41.7207) (-8.5519, 41.7296) (-8.5526, 41.7384) (-8.5533, 41.7473) (-8.5542, 41.7562) (-8.5552, 41.7651) (-8.5562, 41.774) (-8.5574, 41.7829) (-8.5587, 41.792) (-8.5601, 41.8011) (-8.5616, 41.8101) (-8.5632, 41.8193) (-8.565, 41.8286) (-8.567, 41.8378) (-8.5691, 41.8474) (-8.5714, 41.8569) (-8.5739, 41.8664) (-8.5766, 41.8764) (-8.5795, 41.8863) (-8.5827, 41.8961) (-8.5861, 41.9066) (-8.5898, 41.9171) (-8.5938, 41.9274) (-8.5982, 41.9386) (-8.603, 41.9496) (-8.6082, 41.9605) (-8.6139, 41.9725) (-8.62, 41.9843) (-8.6267, 41.9957) (-8.6341, 42.0086) (-8.6421, 42.021) (-8.6508, 42.0331) (-8.6605, 42.0466) (-8.6709, 42.0596) (-8.682, 42.072) (-8.6945, 42.0859) (-8.708, 42.0991) (-8.7222, 42.1113) (-8.7379, 42.1248) (-8.7547, 42.1372) (-8.7723, 42.1483) (-8.7914, 42.1604) (-8.8114, 42.171) (-8.8322, 42.1797) (-8.8521, 42.188) (-8.8726, 42.1945) (-8.8933, 42.2007) (-8.9954, 42.2314) (-9.0997, 42.2533) (-9.2027, 42.2803) (-9.3057, 42.3072) (-9.4074, 42.3392) (-9.5115, 42.3625) (-9.5325, 42.3672) (-9.5536, 42.3716) (-9.575, 42.3741) (-9.5974, 42.3767) (-9.6201, 42.3772) (-9.6426, 42.376) (-9.6634, 42.375) (-9.6841, 42.3724) (-9.7045, 42.3683) (-9.7229, 42.3646) (-9.741, 42.3598) (-9.7587, 42.3538) (-9.7745, 42.3484) (-9.79, 42.3422) (-9.805, 42.3351) (-9.8185, 42.3288) (-9.8316, 42.3219) (-9.8443, 42.3144) (-9.8558, 42.3076) (-9.8669, 42.3004) (-9.8777, 42.2927) (-9.8876, 42.2858) (-9.8971, 42.2785) (-9.9065, 42.2709) (-9.915, 42.2639) (-9.9234, 42.2566) (-9.9315, 42.2491) (-9.9391, 42.242) (-9.9465, 42.2348) (-9.9537, 42.2274) (-9.9605, 42.2204) (-9.9672, 42.2132) (-9.9737, 42.2059) (-9.98, 42.1988) (-9.986, 42.1916) (-9.992, 42.1844) (-9.9978, 42.1773) (-10.0034, 42.1701) (-10.0089, 42.1628) (-10.0144, 42.1556) (-10.0196, 42.1483) (-10.0248, 42.141) (-10.0299, 42.1337) (-10.035, 42.1263) (-10.0399, 42.1189) (-10.0448, 42.1115) (-10.0496, 42.104) (-10.0542, 42.0965) (-10.059, 42.0889) (-10.0636, 42.0812) (-10.0681, 42.0735) (-10.0726, 42.0658) (-10.0771, 42.058) (-10.0815, 42.0501) (-10.0859, 42.0421) (-10.0902, 42.0341) (-10.0945, 42.026) (-10.0988, 42.0178) (-10.1031, 42.0096) (-10.1072, 42.0013) (-10.1114, 41.9929) (-10.1156, 41.9844) (-10.1197, 41.9759) (-10.1238, 41.9672) (-10.1279, 41.9585) (-10.1319, 41.9497) (-10.136, 41.9408) (-10.14, 41.9318) (-10.1439, 41.9228) (-10.148, 41.9135) (-10.1519, 41.9043) (-10.1558, 41.895) (-10.1734, 41.8536) (-10.1913, 41.8123) (-10.2098, 41.7713) (-10.2238, 41.7403) (-10.2381, 41.7094) (-10.2527, 41.6786) (-10.2689, 41.6443) (-10.2855, 41.6102) (-10.3023, 41.5762) (-10.3209, 41.5387) (-10.3398, 41.5014) (-10.359, 41.4643) (-10.38, 41.4237) (-10.4014, 41.3833) (-10.4232, 41.3431) (-10.4467, 41.2995) (-10.4707, 41.2561) (-10.4951, 41.2129) (-10.5213, 41.1663) (-10.548, 41.1199) (-10.5751, 41.0738) (-10.6042, 41.0244) (-10.6337, 40.9752) (-10.6636, 40.9262) (-10.6956, 40.874) (-10.728, 40.822) (-10.7609, 40.7703) (-10.7958, 40.7154) (-10.8313, 40.6607) (-10.8673, 40.6064) (-10.9053, 40.5489) (-10.9439, 40.4916) (-10.983, 40.4348) (-11.0243, 40.3747) (-11.0662, 40.315) (-11.1086, 40.2556) (-11.1869, 40.1459) (-11.267, 40.0374) (-11.3487, 39.93) knots 0 0 0 0 0.057795 0.057795 0.057795 0.089038 0.089038 0.089038 0.118617 0.118617 0.118617 0.14653 0.14653 0.14653 0.172778 0.172778 0.172778 0.19736 0.19736 0.19736 0.220277 0.220277 0.220277 0.241529 0.241529 0.241529 0.261115 0.261115 0.261115 0.279036 0.279036 0.279036 0.295292 0.295292 0.295292 0.309882 0.309882 0.309882 0.329164 0.329164 0.329164 0.333477 0.333477 0.333477 0.337694 0.337694 0.337694 0.34182 0.34182 0.34182 0.345864 0.345864 0.345864 0.349834 0.349834 0.349834 0.353742 0.353742 0.353742 0.3576 0.3576 0.3576 0.361424 0.361424 0.361424 0.365232 0.365232 0.365232 0.369048 0.369048 0.369048 0.372899 0.372899 0.372899 0.376819 0.376819 0.376819 0.380853 0.380853 0.380853 0.385052 0.385052 0.385052 0.389482 0.389482 0.389482 0.394225 0.394225 0.394225 0.399381 0.399381 0.399381 0.405067 0.405067 0.405067 0.411413 0.411413 0.411413 0.418548 0.418548 0.418548 0.426565 0.426565 0.426565 0.435472 0.435472 0.435472 0.445133 0.445133 0.445133 0.45436 0.45436 0.45436 0.5 0.5 0.5 0.54564 0.54564 0.54564 0.554867 0.554867 0.554867 0.564528 0.564528 0.564528 0.573435 0.573435 0.573435 0.581452 0.581452 0.581452 0.588587 0.588587 0.588587 0.594933 0.594933 0.594933 0.600619 0.600619 0.600619 0.605775 0.605775 0.605775 0.610518 0.610518 0.610518 0.614948 0.614948 0.614948 0.619147 0.619147 0.619147 0.623181 0.623181 0.623181 0.627101 0.627101 0.627101 0.630952 0.630952 0.630952 0.634768 0.634768 0.634768 0.638576 0.638576 0.638576 0.6424 0.6424 0.6424 0.646258 0.646258 0.646258 0.650166 0.650166 0.650166 0.654136 0.654136 0.654136 0.65818 0.65818 0.65818 0.662306 0.662306 0.662306 0.666523 0.666523 0.666523 0.670836 0.670836 0.670836 0.690118 0.690118 0.690118 0.704708 0.704708 0.704708 0.720964 0.720964 0.720964 0.738885 0.738885 0.738885 0.758471 0.758471 0.758471 0.779723 0.779723 0.779723 0.80264 0.80264 0.80264 0.827222 0.827222 0.827222 0.85347 0.85347 0.85347 0.881383 0.881383 0.881383 0.910962 0.910962 0.910962 0.942205 0.942205 0.942205 1 1 1 1
  arc A239 (-8.4829, 39.1802) -> (-7.3471, 38.9457) centre (0.0435, 77.6158) ccw
  spline S38 degree 3 poles (-4.4186, 38.4995) (-4.4511, 38.6303) (-4.4817, 38.7617) (-4.5102, 38.8935) (-4.5256, 38.9648) (-4.5404, 39.0362) (-4.5545, 39.1077) (-4.5679, 39.1754) (-4.5807, 39.2433) (-4.5929, 39.3112) (-4.6044, 39.3753) (-4.6153, 39.4395) (-4.6257, 39.5038) (-4.6354, 39.5643) (-4.6446, 39.6249) (-4.6533, 39.6855) (-4.6614, 39.7423) (-4.669, 39.7991) (-4.6761, 39.8561) (-4.6827, 39.9091) (-4.6888, 39.9623) (-4.6945, 40.0154) (-4.6998, 40.0648) (-4.7046, 40.1141) (-4.709, 40.1635) (-4.713, 40.209) (-4.7167, 40.2546) (-4.7199, 40.3002) (-4.7228, 40.3419) (-4.7254, 40.3836) (-4.7276, 40.4254) (-4.7296, 40.4633) (-4.7313, 40.5012) (-4.7327, 40.5391) (-4.7339, 40.5731) (-4.7348, 40.6072) (-4.7353, 40.6412) (-4.7361, 40.6862) (-4.7362, 40.7312) (-4.7359, 40.7762) (-4.7359, 40.7862) (-4.7358, 40.7963) (-4.7358, 40.8064) (-4.7359, 40.8162) (-4.736, 40.826) (-4.7362, 40.8359) (-4.7364, 40.8455) (-4.7367, 40.8551) (-4.7371, 40.8648) (-4.7374, 40.8742) (-4.7379, 40.8836) (-4.7385, 40.893) (-4.739, 40.9023) (-4.7396, 40.9115) (-4.7403, 40.9208) (-4.7411, 40.9299) (-4.7419, 40.9389) (-4.7428, 40.948) (-4.7437, 40.957) (-4.7447, 40.9659) (-4.7458, 40.9749) (-4.7469, 40.9837) (-4.7481, 40.9925) (-4.7494, 41.0014) (-4.7507, 41.0102) (-4.7522, 41.0189) (-4.7537, 41.0277) (-4.7553, 41.0364) (-4.757, 41.0452) (-4.7588, 41.0539) (-4.7606, 41.0627) (-4.7626, 41.0715) (-4.7648, 41.0802) (-4.7669, 41.0891) (-4.7693, 41.0979) (-4.7718, 41.1067) (-4.7743, 41.1158) (-4.7771, 41.1248) (-4.78, 41.1337) (-4.7831, 41.143) (-4.7864, 41.1523) (-4.7899, 41.1614) (-4.7936, 41.1711) (-4.7975, 41.1807) (-4.8017, 41.1901) (-4.8062, 41.2002) (-4.811, 41.2102) (-4.8161, 41.22) (-4.8216, 41.2307) (-4.8275, 41.2412) (-4.8338, 41.2515) (-4.8407, 41.2628) (-4.8481, 41.2739) (-4.8559, 41.2846) (-4.8646, 41.2966) (-4.8739, 41.3081) (-4.8837, 41.3192) (-4.8948, 41.3317) (-4.9065, 41.3435) (-4.9189, 41.3547) (-4.9328, 41.3672) (-4.9475, 41.3789) (-4.9629, 41.3895) (-4.98, 41.4013) (-4.998, 41.4119) (-5.0167, 41.4211) (-5.0369, 41.4311) (-5.0579, 41.4396) (-5.0795, 41.446) (-5.1001, 41.4522) (-5.1213, 41.4566) (-5.1425, 41.4606) (-5.2472, 41.4804) (-5.3533, 41.4913) (-5.4585, 41.5074) (-5.5638, 41.5234) (-5.6683, 41.5446) (-5.7742, 41.5569) (-5.7956, 41.5593) (-5.817, 41.5615) (-5.8386, 41.5617) (-5.8611, 41.562) (-5.8837, 41.5602) (-5.906, 41.5566) (-5.9266, 41.5534) (-5.9469, 41.5486) (-5.9667, 41.5425) (-5.9846, 41.5369) (-6.0021, 41.5301) (-6.0191, 41.5223) (-6.0343, 41.5154) (-6.049, 41.5075) (-6.0633, 41.4989) (-6.0759, 41.4913) (-6.0883, 41.483) (-6.1002, 41.4742) (-6.1108, 41.4663) (-6.1211, 41.4579) (-6.1311, 41.4492) (-6.1402, 41.4412) (-6.1489, 41.433) (-6.1574, 41.4244) (-6.1652, 41.4166) (-6.1727, 41.4085) (-6.18, 41.4001) (-6.1869, 41.3924) (-6.1935, 41.3844) (-6.1999, 41.3763) (-6.2059, 41.3686) (-6.2118, 41.3607) (-6.2175, 41.3528) (-6.223, 41.3451) (-6.2283, 41.3373) (-6.2334, 41.3295) (-6.2384, 41.3218) (-6.2433, 41.314) (-6.248, 41.3062) (-6.2527, 41.2985) (-6.2572, 41.2907) (-6.2615, 41.2829) (-6.2659, 41.2751) (-6.2701, 41.2673) (-6.2742, 41.2594) (-6.2783, 41.2515) (-6.2823, 41.2435) (-6.2861, 41.2355) (-6.29, 41.2275) (-6.2938, 41.2194) (-6.2975, 41.2113) (-6.3012, 41.2031) (-6.3048, 41.1949) (-6.3084, 41.1866) (-6.3119, 41.1782) (-6.3154, 41.1697) (-6.3188, 41.1613) (-6.3223, 41.1527) (-6.3256, 41.144) (-6.3289, 41.1354) (-6.3322, 41.1265) (-6.3354, 41.1177) (-6.3386, 41.1088) (-6.3418, 41.0997) (-6.345, 41.0906) (-6.348, 41.0815) (-6.3512, 41.0722) (-6.3542, 41.0628) (-6.3572, 41.0534) (-6.3602, 41.0438) (-6.3632, 41.0342) (-6.3661, 41.0246) (-6.3792, 40.9815) (-6.3927, 40.9386) (-6.4068, 40.8959) (-6.4175, 40.8636) (-6.4285, 40.8313) (-6.4398, 40.7992) (-6.4524, 40.7634) (-6.4653, 40.7278) (-6.4785, 40.6922) (-6.493, 40.653) (-6.5079, 40.6139) (-6.5232, 40.575) (-6.5398, 40.5324) (-6.5569, 40.49) (-6.5743, 40.4477) (-6.5932, 40.4019) (-6.6125, 40.3562) (-6.6322, 40.3107) (-6.6535, 40.2616) (-6.6752, 40.2127) (-6.6973, 40.1641) (-6.721, 40.1118) (-6.7452, 40.0598) (-6.7699, 40.008) (-6.7962, 39.9527) (-6.823, 39.8976) (-6.8503, 39.8428) (-6.8793, 39.7845) (-6.9089, 39.7265) (-6.939, 39.6687) (-6.9708, 39.6074) (-7.0032, 39.5465) (-7.0362, 39.4858) (-7.071, 39.4218) (-7.1063, 39.358) (-7.1423, 39.2946) (-7.2087, 39.1772) (-7.2771, 39.0609) (-7.3471, 38.9457) knots 0 0 0 0 0.057795 0.057795 0.057795 0.089038 0.089038 0.089038 0.118617 0.118617 0.118617 0.14653 0.14653 0.14653 0.172778 0.172778 0.172778 0.19736 0.19736 0.19736 0.220277 0.220277 0.220277 0.241529 0.241529 0.241529 0.261115 0.261115 0.261115 0.279036 0.279036 0.279036 0.295292 0.295292 0.295292 0.309882 0.309882 0.309882 0.329164 0.329164 0.329164 0.333477 0.333477 0.333477 0.337694 0.337694 0.337694 0.34182 0.34182 0.34182 0.345864 0.345864 0.345864 0.349834 0.349834 0.349834 0.353742 0.353742 0.353742 0.3576 0.3576 0.3576 0.361424 0.361424 0.361424 0.365232 0.365232 0.365232 0.369048 0.369048 0.369048 0.372899 0.372899 0.372899 0.376819 0.376819 0.376819 0.380853 0.380853 0.380853 0.385052 0.385052 0.385052 0.389482 0.389482 0.389482 0.394225 0.394225 0.394225 0.399381 0.399381 0.399381 0.405067 0.405067 0.405067 0.411413 0.411413 0.411413 0.418548 0.418548 0.418548 0.426565 0.426565 0.426565 0.435472 0.435472 0.435472 0.445133 0.445133 0.445133 0.45436 0.45436 0.45436 0.5 0.5 0.5 0.54564 0.54564 0.54564 0.554867 0.554867 0.554867 0.564528 0.564528 0.564528 0.573435 0.573435 0.573435 0.581452 0.581452 0.581452 0.588587 0.588587 0.588587 0.594933 0.594933 0.594933 0.600619 0.600619 0.600619 0.605775 0.605775 0.605775 0.610518 0.610518 0.610518 0.614948 0.614948 0.614948 0.619147 0.619147 0.619147 0.623181 0.623181 0.623181 0.627101 0.627101 0.627101 0.630952 0.630952 0.630952 0.634768 0.634768 0.634768 0.638576 0.638576 0.638576 0.6424 0.6424 0.6424 0.646258 0.646258 0.646258 0.650166 0.650166 0.650166 0.654136 0.654136 0.654136 0.65818 0.65818 0.65818 0.662306 0.662306 0.662306 0.666523 0.666523 0.666523 0.670836 0.670836 0.670836 0.690118 0.690118 0.690118 0.704708 0.704708 0.704708 0.720964 0.720964 0.720964 0.738885 0.738885 0.738885 0.758471 0.758471 0.758471 0.779723 0.779723 0.779723 0.80264 0.80264 0.80264 0.827222 0.827222 0.827222 0.85347 0.85347 0.85347 0.881383 0.881383 0.881383 0.910962 0.910962 0.910962 0.942205 0.942205 0.942205 1 1 1 1
  arc A240 (-4.4186, 38.4995) -> (-3.2645, 38.385) centre (0.0435, 77.6158) ccw